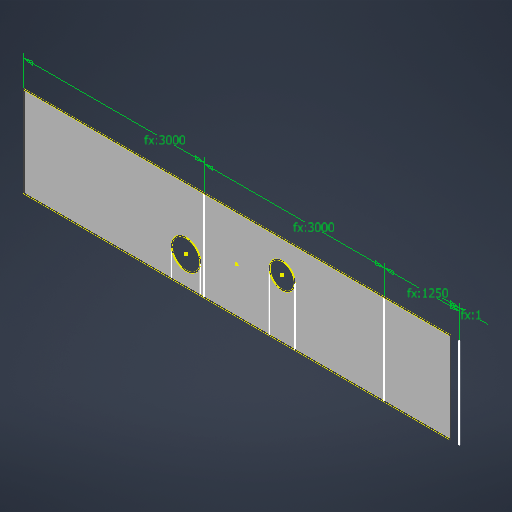
# Autodesk Inventor part: Sheet divider
Saved by Autodesk Inventor 2027 (Build 310192000, 192)
## iProperties
RuleStatus: InUse
Created: 2026-05-15
Part Number: Sheet divider
Material: Generic
Document SubType Name: Sheet Metal
Designer: Jelte
Density: 1 g/cm^3
Sheet Metal Rule: Default
Appearance: Default
Flat Pattern Width: 150 cm
Flat Pattern Length: 710 cm
Flat Pattern Area: 106500 cm^2
Sheet Metal Width: 1500,000 mm
Sheet Metal Length: 7100,000 mm
Sheet Metal Area: 10650000,000 mm^2
Author: Jelte
Autodesk Inventor part; units mm, degrees
note: some values were not read from the file. Left out: dimensions or parameters whose unit could not be read.
ref_plane "YZ Plane" through (0, 0, 0) normal (1, 0, 0) x (0, 1, 0)
ref_plane "XZ Plane" through (0, 0, 0) normal (0, 1, 0) x (-1, 0, 0)
ref_plane "XY Plane" through (0, 0, 0) normal (0, 0, 1) x (1, 0, 0)
sketch "Sketch1" plane through (0, 0, 0) normal (0, 0, 1) x (1, 0, 0)
  line L0 (3550, -750) -> (-3550, -750)
  line L1 (-3550, -750) -> (-3550, 750)
  line L2 (-3550, 750) -> (3550, 750)
  line L3 (3550, 750) -> (3550, -750)
  line L4 (3550, -750) -> (-3550, 750) construction
  line L5 (-3550, -750) -> (3550, 750) construction
  point P0 (0, 0)
  dimension "d6" = 7100
  measures "d6" distance of L1.end L2.end
extrude "Plate1" add sketch "Sketch1" along normal blind 3.048
sketch "Sketch2" plane through (0, 0, 3.048) normal (0, 0, 1) x (1, 0, 0)
  circle A0 centre (750, 214.837) radius 210
  circle A1 centre (-850, -278.831) radius 240
  line L0 (-3550, -750) -> (-3550, 750) projected
  point P0 (0, 0)
  dimension "d2" = 4300
  dimension "d3" = 2700
  dimension "d11" = 420
  dimension "d12" = 480
  constraints: 2 centre point
  measures "d2" distance from line of A0.centre L0
  measures "d3" distance from line of A1.centre L0
  measures "d11" diameter of A0
  measures "d12" diameter of A1
extrude "Cut1" cut sketch "Sketch2" against normal blind 3.048
sketch "Sketch3" plane through (0, 0, 3.048) normal (0, 0, 1) x (1, 0, 0)
  line L0 (3550, 750) -> (-3550, 750) projected
  line L1 (-550, 750) -> (-550, -750)
  line L2 (-3550, -750) -> (3550, -750) projected
  line L3 (2450, 750) -> (2450, -750)
  line L4 (3700, -750) -> (3700, 750)
  line L5 (-3550, -750) -> (-3550, 750) projected
  line L6 (3701, 750) -> (3701, -750)
  circle A0 centre (750, 214.837) radius 210 projected
  line L7 (540, 214.837) -> (540, -750)
  line L8 (960, 214.837) -> (960, -750)
  circle A1 centre (-850, -278.831) radius 240 projected
  line L9 (-610, -278.831) -> (-610, -750)
  line L10 (-1090, -278.831) -> (-1090, -750)
  point P0 (0, 0)
  dimension "d7" = 3000
  dimension "d8" = 3000
  dimension "d9" = 1250
  dimension "d10" = 1
  constraints: 16 end point, 7 vertical, 4 point on circle, 4 tangent, 3 point on line, 1 perpendicular, 8 other
  measures "d7" distance between parallel lines of L1 L5
  measures "d8" distance between parallel lines of L3 L1
  measures "d9" distance between parallel lines of L4 L3
  measures "d10" distance between parallel lines of L6 L4
equation "\"d6\" = Length"
equation "\"d2\" = Hole1"
equation "\"d3\" = Hole2"
equation "\"d4\" = Thickness"
equation "\"d7\" = S1"
equation "\"d8\" = S2"
equation "\"d9\" = S3"
equation "\"d10\" = S4"
equation "\"d1\" = Thickness"
equation "\"BendRadius\" = Thickness"
equation "\"BendReliefWidth\" = Thickness"
equation "\"BendReliefDepth\" = 0.5 * Thickness"
equation "\"CornerReliefSize\" = 4 * Thickness"
equation "\"MinimumRemnant\" = 2 * Thickness"
equation "\"TransitionRadius\" = BendRadius"
equation "\"JacobiRadiusSize\" = BendRadius"
equation "\"GapSize\" = Thickness"
equation "\"Length\" = 7100"
equation "\"Hole1\" = 4300"
equation "\"Hole2\" = 2700"
equation "\"S1\" = 3000"
equation "\"S2\" = 3000"
equation "\"S3\" = 1250"
equation "\"S4\" = 1"
equation "\"Thickness\" = 3.048"
body "Solid1"
